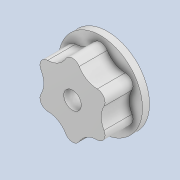
# Autodesk Inventor part: 原動節接続部v2内-1
Saved by Autodesk Inventor 2020.4 (Build 244396000, 396)
## iProperties
Created: 2021-02-21
Part Number: 原動節接続部v2内-1
Material: アルミニウム 2014-T4
Document SubType Name: Modeling
Designer: AA19065
Density: 2.8 g/cm^3
Appearance: サテン
Mass: 0.995673 g
Surface Area: 4.24036 cm^2
Volume: 0.355598 cm^3
Author: AA19065
Autodesk Inventor part; units mm, degrees
ref_plane "YZ Plane" through (0, 0, 0) normal (1, 0, 0) x (0, 1, 0)
ref_plane "XZ Plane" through (0, 0, 0) normal (0, 1, 0) x (-1, 0, 0)
ref_plane "XY Plane" through (0, 0, 0) normal (0, 0, 1) x (1, 0, 0)
sketch "スケッチ1" plane through (0, 0, 0) normal (0, 0, 1) x (1, 0, 0)
  arc A0 (-16.2703, -9.5731) -> (-13.6889, -8.0827) centre (-16.2703, -6.5923) ccw
  arc A1 (-16.2703, -9.5731) -> (-17.2313, -10.1279) centre (-16.2703, -10.6827) ccw
  arc A2 (-17.2313, -10.1279) -> (-17.2313, -11.2375) centre (-16.2703, -10.6827) ccw
  arc A3 (-17.2313, -14.2183) -> (-17.2313, -11.2375) centre (-19.8127, -12.7279) ccw
  arc A4 (-17.2313, -14.2183) -> (-17.2313, -15.3279) centre (-16.2703, -14.7731) ccw
  arc A5 (-17.2313, -15.3279) -> (-16.2703, -15.8827) centre (-16.2703, -14.7731) ccw
  arc A6 (-13.6889, -17.3731) -> (-16.2703, -15.8827) centre (-16.2703, -18.8635) ccw
  arc A7 (-13.6889, -17.3731) -> (-12.7279, -17.9279) centre (-12.7279, -16.8183) ccw
  arc A8 (-12.7279, -17.9279) -> (-11.767, -17.3731) centre (-12.7279, -16.8183) ccw
  arc A9 (-9.1855, -15.8827) -> (-11.767, -17.3731) centre (-9.1855, -18.8635) ccw
  arc A10 (-9.1855, -15.8827) -> (-8.2246, -15.3279) centre (-9.1855, -14.7731) ccw
  arc A11 (-8.2246, -15.3279) -> (-8.2246, -14.2183) centre (-9.1855, -14.7731) ccw
  arc A12 (-8.2246, -11.2375) -> (-8.2246, -14.2183) centre (-5.6431, -12.7279) ccw
  arc A13 (-8.2246, -11.2375) -> (-8.2246, -10.1279) centre (-9.1855, -10.6827) ccw
  arc A14 (-8.2246, -10.1279) -> (-9.1855, -9.5731) centre (-9.1855, -10.6827) ccw
  arc A15 (-11.767, -8.0827) -> (-9.1855, -9.5731) centre (-9.1855, -6.5923) ccw
  arc A16 (-11.767, -8.0827) -> (-12.7279, -7.5279) centre (-12.7279, -8.6375) ccw
  arc A17 (-12.7279, -7.5279) -> (-13.6889, -8.0827) centre (-12.7279, -8.6375) ccw
  circle A18 centre (-12.7279, -12.7279) radius 1.5 construction
  circle A19 centre (-12.7279, -12.7279) radius 1.25
  circle A20 centre (-12.7279, -12.7279) radius 6
  point P0 (0, 0)
  point P1 (0, 0)
  dimension "d0" = 2.5
  constraints: 36 point on circle, 21 centre point, 1 coincident, 20 other
  measures "d0" diameter of A19
extrude "押し出し1" add sketch "スケッチ1" against normal blind 1 contours A0 A17 A16 A15 A14 A13 A12 A11 A10 A9 A8 A7 A6 A5 A4 A3 A2 A1 | A20
extrude "押し出し2" add sketch "スケッチ1" along normal blind 4 contours A0 A17 A16 A15 A14 A13 A12 A11 A10 A9 A8 A7 A6 A5 A4 A3 A2 A1
sketch "書き出し" plane through (0, 0, 4) normal (0, 0, 1) x (1, 0, 0)
  arc A0 (-13.6889, -17.3731) -> (-11.767, -17.3731) centre (-12.7279, -16.8183) ccw projected
  arc A1 (-9.1855, -15.8827) -> (-11.767, -17.3731) centre (-9.1855, -18.8635) ccw projected
  arc A2 (-9.1855, -15.8827) -> (-8.2246, -14.2183) centre (-9.1855, -14.7731) ccw projected
  arc A3 (-8.2246, -11.2375) -> (-8.2246, -14.2183) centre (-5.6431, -12.7279) ccw projected
  arc A4 (-8.2246, -11.2375) -> (-9.1855, -9.5731) centre (-9.1855, -10.6827) ccw projected
  arc A5 (-11.767, -8.0827) -> (-9.1855, -9.5731) centre (-9.1855, -6.5923) ccw projected
  arc A6 (-11.767, -8.0827) -> (-13.6889, -8.0827) centre (-12.7279, -8.6375) ccw projected
  arc A7 (-16.2703, -9.5731) -> (-13.6889, -8.0827) centre (-16.2703, -6.5923) ccw projected
  arc A8 (-16.2703, -9.5731) -> (-17.2313, -11.2375) centre (-16.2703, -10.6827) ccw projected
  arc A9 (-17.2313, -14.2183) -> (-17.2313, -11.2375) centre (-19.8127, -12.7279) ccw projected
  arc A10 (-17.2313, -14.2183) -> (-16.2703, -15.8827) centre (-16.2703, -14.7731) ccw projected
  arc A11 (-13.6889, -17.3731) -> (-16.2703, -15.8827) centre (-16.2703, -18.8635) ccw projected
  circle A12 centre (-12.7279, -12.7279) radius 1.25 projected
  arc A13 (-13.6889, -17.3731) -> (-16.2703, -15.8827) centre (-16.2703, -18.8635) ccw projected
  arc A14 (-17.2313, -14.2183) -> (-16.2703, -15.8827) centre (-16.2703, -14.7731) ccw projected
  arc A15 (-17.2313, -14.2183) -> (-17.2313, -11.2375) centre (-19.8127, -12.7279) ccw projected
  arc A16 (-16.2703, -9.5731) -> (-17.2313, -11.2375) centre (-16.2703, -10.6827) ccw projected
  arc A17 (-16.2703, -9.5731) -> (-13.6889, -8.0827) centre (-16.2703, -6.5923) ccw projected
  arc A18 (-11.767, -8.0827) -> (-13.6889, -8.0827) centre (-12.7279, -8.6375) ccw projected
  arc A19 (-11.767, -8.0827) -> (-9.1855, -9.5731) centre (-9.1855, -6.5923) ccw projected
  arc A20 (-8.2246, -11.2375) -> (-9.1855, -9.5731) centre (-9.1855, -10.6827) ccw projected
  arc A21 (-8.2246, -11.2375) -> (-8.2246, -14.2183) centre (-5.6431, -12.7279) ccw projected
  arc A22 (-9.1855, -15.8827) -> (-8.2246, -14.2183) centre (-9.1855, -14.7731) ccw projected
  arc A23 (-9.1855, -15.8827) -> (-11.767, -17.3731) centre (-9.1855, -18.8635) ccw projected
  arc A24 (-13.6889, -17.3731) -> (-11.767, -17.3731) centre (-12.7279, -16.8183) ccw projected
  circle A25 centre (-12.7279, -12.7279) radius 6 projected
  circle A26 centre (-12.7279, -12.7279) radius 7.5
  point P0 (0, 0)
  dimension "d5" = 1.5
  constraints: 1 centre point
  measures "d5" radial gap between concentric circles of A25 A26
